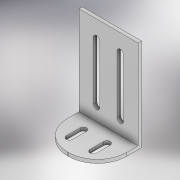
# Autodesk Inventor part: Vertical_L_Bracket
Saved by Autodesk Inventor 2020.3 (Build 243373000, 373)
## iProperties
Created: 2021-08-03
Part Number: Vertical_L_Bracket
Material: Aluminum 6061
Document SubType Name: Modeling
Designer: justi
Density: 2.7 g/cm^3
Appearance: Aluminum - Dark
Author: justi
Autodesk Inventor part; units mm, degrees
ref_plane "YZ Plane" through (0, 0, 0) normal (1, 0, 0) x (0, 1, 0)
ref_plane "XZ Plane" through (0, 0, 0) normal (0, 1, 0) x (-1, 0, 0)
ref_plane "XY Plane" through (0, 0, 0) normal (0, 0, 1) x (1, 0, 0)
sketch "Sketch2" plane through (0, 0, 0) normal (0, 0, 1) x (1, 0, 0)
  line L0 (-25.5, 40) -> (25.5, 40)
  line L1 (25.5, 40) -> (25.5, -40)
  line L2 (25.5, -40) -> (-25.5, -40)
  line L3 (-25.5, -40) -> (-25.5, 40)
  line L4 (-25.5, 40) -> (25.5, -40) construction
  line L5 (25.5, 40) -> (-25.5, -40) construction
  line L6 (-25.5, 0) -> (-10.25, 0) construction
  line L7 (25.5, 0) -> (10.25, 0) construction
  line L8 (-10.25, -25) -> (-10.25, 25) construction
  line L9 (-7.5, -25) -> (-7.5, 25)
  line L10 (-13, 25) -> (-13, -25)
  arc A0 (-13, -25) -> (-7.5, -25) centre (-10.25, -25) ccw
  arc A1 (-7.5, 25) -> (-13, 25) centre (-10.25, 25) ccw
  line L11 (10.25, -25) -> (10.25, 25) construction
  line L12 (13, -25) -> (13, 25)
  line L13 (7.5, 25) -> (7.5, -25)
  arc A2 (7.5, -25) -> (13, -25) centre (10.25, -25) ccw
  arc A3 (13, 25) -> (7.5, 25) centre (10.25, 25) ccw
  point P0 (0, 0)
  dimension "d2" = 51
  dimension "d3" = 80
  dimension "d4" = 15.25
  dimension "d5" = 15.25
  dimension "d6" = 25
  dimension "d7" = 5.5
  dimension "d8" = 25
  dimension "d9" = 5.5
  constraints: 32 end point, 8 point on circle, 8 tangent, 6 midpoint, 4 centre point, 4 parallel, 3 horizontal, 2 perpendicular, 1 vertical
  measures "d2" distance of L1.end L2.end
  measures "d3" distance of L0.end L1.end
  measures "d4" distance of L6.start L6.end
  measures "d5" distance of L7.start L7.end
  measures "d6" distance of L6.end L8.end
  measures "d7" diameter of A1
  measures "d8" distance of L7.end L11.end
  measures "d9" diameter of A3
extrude "Extrusion1" add sketch "Sketch2" along normal blind 3
sketch "Sketch3" plane through (0, 0, 3) normal (0, 0, 1) x (1, 0, 0)
  line L0 (25.5, -40) -> (25.5, 40) projected
  line L1 (-25.5, -40) -> (25.5, -40)
  line L2 (25.5, -40) -> (25.5, -37)
  line L3 (25.5, -37) -> (-25.5, -37)
  line L4 (-25.5, -37) -> (-25.5, -40)
  point P0 (0, 0)
  dimension "d12" = 3
  constraints: 8 end point, 2 parallel, 1 horizontal, 1 perpendicular, 1 point on line
  measures "d12" distance of L2.end L1.end
extrude "Extrusion2" add sketch "Sketch3" along normal blind 35
sketch "Sketch4" plane through (-25.5, -37, 3) normal (0, 1, 0) x (1, 0, 0)
  line L0 (0, 0) -> (51, 0) construction
  line L1 (25.5, 0) -> (25.5, -35) construction
  line L2 (51, -35) -> (0, -35) construction
  line L3 (0, 3) -> (0, -35) construction
  line L4 (0, -17.5) -> (15.25, -17.5) construction
  line L5 (0, -17.5) -> (15.25, -17.5) construction
  line L6 (51, 0) -> (51, -35) construction
  line L7 (51, -17.5) -> (35.75, -17.5) construction
  line L8 (15.25, -23.5) -> (15.25, -11.5) construction
  line L9 (18, -23.5) -> (18, -11.5)
  line L10 (12.5, -11.5) -> (12.5, -23.5)
  arc A0 (12.5, -23.5) -> (18, -23.5) centre (15.25, -23.5) ccw
  arc A1 (18, -11.5) -> (12.5, -11.5) centre (15.25, -11.5) ccw
  line L11 (35.75, -23.5) -> (35.75, -11.5) construction
  line L12 (38.5, -23.5) -> (38.5, -11.5)
  line L13 (33, -11.5) -> (33, -23.5)
  arc A2 (33, -23.5) -> (38.5, -23.5) centre (35.75, -23.5) ccw
  arc A3 (38.5, -11.5) -> (33, -11.5) centre (35.75, -11.5) ccw
  point P0 (25.5, 3)
  dimension "d15" = 15.25
  dimension "d17" = 15.25
  dimension "d18" = 6
  dimension "d19" = 5.5
  dimension "d20" = 6
  dimension "d21" = 5.5
  constraints: 24 end point, 8 point on circle, 8 tangent, 5 midpoint, 4 centre point, 2 horizontal, 2 parallel, 2 perpendicular, 1 collinear, 1 point on line, 1 vertical
  measures "d15" distance of L4.start L4.end
  measures "d17" distance of L7.start L7.end
  measures "d18" distance of L5.end L8.end
  measures "d19" diameter of A1
  measures "d20" distance of L7.end L11.end
  measures "d21" diameter of A3
extrude "Extrusion3" cut sketch "Sketch4" against normal through all
fillet "Fillet2" radius 25 2 edges at (-25.5, -38.5, 38) (25.5, -38.5, 38)
body "Solid1"
